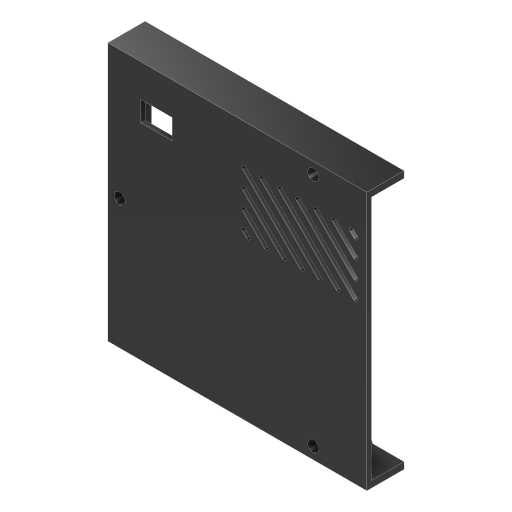
# Autodesk Inventor part: display_cover_part2_back
Saved by Autodesk Inventor 2023 (Build 270158000, 158)
## iProperties
Created: 2024-12-15
Part Number: display_cover_part2_back
Material: Všeobecné
Document SubType Name: Modeling
Designer: Marek
Density: 1 g/cm^3
Appearance: Lesklá – černá
Author: Marek
## iProperties of the stored document display_cover_part2_back_3D tisk.ipt
Created: 2025-01-08
Part Number: display_cover_part2_back_3D tisk
Material: Všeobecné
Document SubType Name: Modeling
Designer: Marek
Density: 1 g/cm^3
Appearance: Výchozí
Author: Marek
Autodesk Inventor part; units mm, degrees
ref_plane "YZ Plane" through (0, 0, 0) normal (1, 0, 0) x (0, 1, 0)
ref_plane "XZ Plane" through (0, 0, 0) normal (0, 1, 0) x (-1, 0, 0)
ref_plane "XY Plane" through (0, 0, 0) normal (0, 0, 1) x (1, 0, 0)
sketch "Náčrt1" plane through (0, 0, 0) normal (0, 0, 1) x (1, 0, 0)
  line L0 (0, 110.95) -> (0, -110.95) projected
  line L1 (-115.25, 0) -> (107, 0) projected
  line L2 (-83.5, 79.25) -> (75.25, 79.25)
  line L3 (75.25, 79.25) -> (75.25, -79.25)
  line L4 (75.25, -79.25) -> (-83.5, -79.25)
  line L5 (-83.5, -79.25) -> (-83.5, 79.25)
  point P0 (0, 0)
  dimension "d0" = 158.75
  dimension "d1" = 158.5
  dimension "d2" = 83.5
  constraints: 8 end point, 2 parallel, 1 horizontal, 1 perpendicular, 1 other
  measures "d0" distance between parallel lines of L5 L3
  measures "d1" distance between parallel lines of L4 L2
  measures "d2" distance between parallel lines of L5 L0
extrude "Vysunutí1" add sketch "Náčrt1" along normal blind 2.8
sketch "Náčrt2" plane through (0, 0, 0) normal (0, 0, -1) x (-1, 0, 0)
  line L0 (0, -110.95) -> (0, 110.95) projected
  line L1 (-107.3, 0) -> (115.3, 0) projected
  line L2 (83.5, -79.25) -> (-75.25, -79.25) projected
  line L3 (83.5, 79.25) -> (83.5, -79.25) projected
  line L4 (-75.25, 79.25) -> (83.5, 79.25) projected
  line L5 (-75.25, -79.25) -> (-75.25, 79.25) projected
  line L6 (-75.25, 75.25) -> (79.5, 75.25)
  line L7 (79.5, 75.25) -> (79.5, -75.25)
  line L8 (79.5, -75.25) -> (-75.25, -75.25)
  line L9 (-75.25, -75.25) -> (-75.25, 75.25)
  line L10 (83.5, -79.25) -> (-75.25, -79.25) projected
  line L11 (-75.25, 79.25) -> (83.5, 79.25)
  line L12 (83.5, 79.25) -> (83.5, -79.25)
  line L13 (83.5, -79.25) -> (-75.25, -79.25)
  line L14 (-75.25, -79.25) -> (-75.25, 79.25)
  line L15 (83.5, 79.25) -> (83.5, -79.25) projected
  arc A0 (79.5, 13.6771) -> (79.5, -13.6771) centre (83.5, 0) ccw
  line L16 (-75.25, 79.25) -> (83.5, 79.25) projected
  arc A1 (-56.0271, 75.25) -> (-28.6729, 75.25) centre (-42.35, 79.25) ccw
  arc A2 (-28.6729, -75.25) -> (-56.0271, -75.25) centre (-42.35, -79.25) ccw
  point P0 (0, 0)
  dimension "d5" = 4
  dimension "d6" = 4
  dimension "d7" = 4
  dimension "d8" = 28.5
  dimension "d9" = 28.5
  dimension "d10" = 28.5
  dimension "d11" = 42.35
  dimension "d12" = 42.35
  constraints: 16 end point, 9 point on line, 6 point on circle, 4 parallel, 3 centre point, 2 horizontal, 2 perpendicular, 1 midpoint
  measures "d5" distance between parallel lines of L4 L6
  measures "d6" distance between parallel lines of L3 L7
  measures "d7" distance between parallel lines of L2 L8
  measures "d8" diameter of A0
  measures "d9" diameter of A1
  measures "d10" diameter of A2
  measures "d11" distance from line of L0 A1.centre
  measures "d12" distance from line of A2.centre L0
extrude "Vysunutí2" add sketch "Náčrt2" along normal blind 20 contours L2 L5 L8 L0 | L0 L8 L7 L1 L3 L2 | L8 A2 | L1 L7 L6 L0 L4 L3 | L6 L5 L4 L0 | A0 L7 L1 | L1 L7 A0 | A1 L6
sketch "Náčrt3" plane through (0, 0, 2.8) normal (0, 0, 1) x (1, 0, 0)
  line L0 (-83.5, -79.25) -> (75.25, -79.25) projected
  line L1 (75.25, -79.25) -> (75.25, 79.25) projected
  line L2 (75.25, 79.25) -> (-83.5, 79.25) projected
  line L3 (-83.5, 79.25) -> (-83.5, -79.25) projected
  line L4 (-115.3, 0) -> (107.3, 0) projected
  line L5 (0, 110.95) -> (0, -110.95) projected
  arc A0 (23.2826, 17.8214) -> (25.4034, 19.9432) centre (24.343, 18.8823) ccw
  line L6 (-1.08, 53.1695) -> (34.2839, 17.8227)
  line L7 (36.4053, 17.8233) -> (-1.0805, 55.2908) construction
  line L8 (36.4047, 19.9446) -> (1.0408, 55.2914)
  arc A1 (34.2839, 17.8227) -> (36.4047, 19.9446) centre (35.3443, 18.8837) ccw
  arc A2 (45.2853, 17.8241) -> (47.4061, 19.9459) centre (46.3457, 18.885) ccw
  line L9 (20.9227, 53.1722) -> (56.2866, 17.8254)
  line L10 (58.4074, 19.9472) -> (23.0435, 55.294)
  line L11 (58.4079, 17.8259) -> (20.9222, 55.2935) construction
  line L12 (31.9396, 53.158) -> (67.0452, 18.0694)
  line L13 (69.166, 20.1912) -> (34.0604, 55.2798)
  line L14 (69.1665, 18.0699) -> (31.9227, 55.2956) construction
  arc A3 (56.2866, 17.8254) -> (58.4074, 19.9472) centre (57.347, 18.8863) ccw
  arc A4 (67.0452, 18.0694) -> (69.166, 20.1912) centre (68.1056, 19.1303) ccw
  line L15 (47.4066, 17.8246) -> (9.9209, 55.2922) construction
  line L16 (9.9214, 53.1709) -> (45.2853, 17.8241)
  arc A5 (12.0422, 55.2927) -> (9.9214, 53.1709) centre (10.9818, 54.2318) ccw
  line L17 (47.4061, 19.9459) -> (12.0422, 55.2927)
  line L18 (53.9267, 53.1762) -> (67.0452, 40.064)
  line L19 (67.2866, 28.8254) -> (42.9254, 53.1748)
  line L20 (69.4079, 28.8259) -> (42.9248, 55.2962) construction
  line L21 (45.0462, 55.2967) -> (69.4074, 30.9472)
  line L22 (69.166, 42.1859) -> (56.0475, 55.298)
  arc A6 (67.2866, 28.8254) -> (69.4074, 30.9472) centre (68.347, 29.8863) ccw
  arc A7 (1.0408, 55.2914) -> (-1.08, 53.1695) centre (-0.0196, 54.2304) ccw
  arc A8 (23.0435, 55.294) -> (20.9227, 53.1722) centre (21.9831, 54.2331) ccw
  line L23 (25.4034, 19.9432) -> (1.0422, 44.2927)
  line L24 (25.4039, 17.8219) -> (-1.0791, 44.2922) construction
  line L25 (-1.0786, 42.1709) -> (23.2826, 17.8214)
  arc A9 (1.0422, 44.2927) -> (-1.0786, 42.1709) centre (-0.0182, 43.2318) ccw
  line L26 (67.2839, 50.8227) -> (64.9396, 53.1659)
  line L27 (67.0604, 55.2878) -> (69.4047, 52.9446)
  line L28 (69.4053, 50.8233) -> (64.9227, 55.3036) construction
  line L29 (69.1665, 40.0645) -> (53.9262, 55.2975) construction
  arc A10 (56.0475, 55.298) -> (53.9267, 53.1762) centre (54.9871, 54.2371) ccw
  arc A11 (12.2813, 17.8201) -> (14.4021, 19.9419) centre (13.3417, 18.881) ccw
  line L30 (14.4021, 19.9419) -> (1.0435, 33.294)
  line L31 (14.4026, 17.8206) -> (-1.0778, 33.2935) construction
  line L32 (-1.0773, 31.1722) -> (12.2813, 17.8201)
  arc A12 (1.0435, 33.294) -> (-1.0773, 31.1722) centre (-0.0169, 32.2331) ccw
  arc A13 (67.2839, 50.8227) -> (69.4047, 52.9446) centre (68.3443, 51.8837) ccw
  arc A14 (45.0462, 55.2967) -> (42.9254, 53.1748) centre (43.9858, 54.2358) ccw
  arc A15 (67.0452, 40.064) -> (69.166, 42.1859) centre (68.1056, 41.125) ccw
  line L33 (1.0448, 22.2953) -> (3.4007, 19.9406)
  arc A16 (1.2799, 17.8187) -> (3.4007, 19.9406) centre (2.3403, 18.8797) ccw
  arc A17 (1.0448, 22.2953) -> (-1.076, 20.1735) centre (-0.0156, 21.2344) ccw
  line L34 (3.4013, 17.8193) -> (-1.0765, 22.2948) construction
  line L35 (1.2799, 17.8187) -> (-1.076, 20.1735)
  arc A18 (34.0604, 55.2798) -> (31.9396, 53.158) centre (33, 54.2189) ccw
  arc A19 (67.0604, 55.2878) -> (64.9396, 53.1659) centre (66, 54.2269) ccw
  point P0 (0, 0)
  dimension "d48" = 3
  dimension "d49" = 3
  dimension "d50" = 3
  dimension "d51" = 3
  dimension "d53" = 3
  dimension "d54" = 3
  dimension "d55" = 3
  dimension "d56" = 3
  dimension "d57" = 3
  dimension "d101" = 23.3345
  dimension "d102" = 31.1127
  dimension "d103" = 38.8909
  dimension "d104" = 46.669
  dimension "d105" = 54.4472
  dimension "d106" = 62.2254
  dimension "d107" = 70.0036
  dimension "d108" = 15.5564
  dimension "d109" = 7.7782
  dimension "d110" = 10.657
  dimension "d131" = 33
  dimension "d132" = 1.5
  dimension "d133" = 66
  dimension "d134" = 1.5
  dimension "d139" = 135.014
  dimension "d140" = 18.5563
  dimension "d141" = 31.1127
  dimension "d142" = 9.157
  dimension "d143" = 1.3789
  dimension "d144" = 50.4241
  dimension "d145" = 28.4267
  dimension "d146" = 39.1855
  dimension "d147" = 23.9464
  dimension "d148" = 61.4254
  dimension "d149" = 61.4267
  dimension "d150" = 23.9544
  dimension "d151" = 61.4281
  dimension "d152" = 61.4294
  dimension "d153" = 23.9573
  dimension "d154" = 61.4307
  dimension "d155" = 56.9547
  dimension "d156" = 45.956
  dimension "d157" = 34.9573
  dimension "d158" = 23.9586
  constraints: 80 end point, 58 point on circle, 37 tangent, 20 centre point, 20 point on line, 12 parallel, 1 equal radius
  measures "d48" distance between parallel lines of L6 L8
  measures "d49" distance between parallel lines of L17 L16
  measures "d50" distance between parallel lines of L25 L23
  measures "d51" distance between parallel lines of L32 L30
  measures "d53" distance between parallel lines of L10 L9
  measures "d54" distance between parallel lines of L12 L13
  measures "d55" distance between parallel lines of L21 L19
  measures "d56" distance between parallel lines of L18 L22
  measures "d57" distance between parallel lines of L26 L27
  measures "d101" distance between parallel lines of L14 L28
  measures "d102" distance between parallel lines of L28 L11
  measures "d103" distance between parallel lines of L28 L15
  measures "d104" distance between parallel lines of L28 L7
  measures "d105" distance between parallel lines of L28 L24
  measures "d106" distance between parallel lines of L28 L31
  measures "d107" distance between parallel lines of L34 L28
  measures "d108" distance between parallel lines of L13 L22
  measures "d109" distance between parallel lines of L29 L20
  measures "d110" distance from line of L4.end L27
  measures "d131" distance from line of L5 A18.centre
  measures "d132" radius of A18
  measures "d133" distance from line of L5 A19.centre
  measures "d134" radius of A19
  measures "d139" angle of L2 L27
  measures "d140" distance between parallel lines of L27 L19
  measures "d141" distance between parallel lines of L27 L10
  measures "d142" distance from line of L4.end L28
  measures "d143" distance from line of L4.end L29
  measures "d144" distance from line of L20.start L2
  measures "d145" distance from line of L28.start L2
  measures "d146" distance from line of L29.start L2
  measures "d147" distance from line of L28.end L2
  measures "d148" distance from line of L15.start L2
  measures "d149" distance from line of L7.start L2
  measures "d150" distance from line of L14.end L2
  measures "d151" distance from line of L24.start L2
  measures "d152" distance from line of L31.start L2
  measures "d153" distance from line of L17.end L2
  measures "d154" distance from line of L34.start L2
  measures "d155" distance from line of L33.start L2
  measures "d156" distance from line of L30.end L2
  measures "d157" distance from line of L23.end L2
  measures "d158" distance from line of L8.end L2
extrude "Vysunutí3" cut sketch "Náčrt3" against normal up to next contours L35 A17 L5 | L5 A17 L33 A16 L35 | A7 L8 A1 L6 L5 | L5 L6 A7 | L32 A12 L5 | L5 A12 L30 A11 L32 | A9 L23 A0 L25 L5 | L5 L25 A9 | L16 A5 L17 A2 | A8 L10 A3 L9 | A18 L13 A4 L12 | A10 L22 A15 L18 | L19 A14 L21 A6 | L26 A19 L27 A13
sketch "Náčrt4" plane through (0, 0, 2.8) normal (0, 0, 1) x (1, 0, 0)
  arc A0 (23.0435, 55.294) -> (20.9227, 53.1722) centre (21.9831, 54.2331) ccw projected
  line L0 (23.0435, 55.294) -> (58.4074, 19.9472) projected
  arc A1 (56.2866, 17.8254) -> (58.4074, 19.9472) centre (57.347, 18.8863) ccw projected
  line L1 (56.2866, 17.8254) -> (20.9227, 53.1722) projected
  arc A2 (67.2839, 50.8227) -> (69.4047, 52.9446) centre (68.3443, 51.8837) ccw projected
  line L2 (67.2839, 50.8227) -> (64.9396, 53.1659) projected
  arc A3 (67.0604, 55.2878) -> (64.9396, 53.1659) centre (66, 54.2269) ccw projected
  line L3 (67.0604, 55.2878) -> (69.4047, 52.9446) projected
  line L4 (1.2799, 17.8187) -> (-1.076, 20.1735) projected
  arc A4 (1.0448, 22.2953) -> (-1.076, 20.1735) centre (-0.0156, 21.2344) ccw projected
  line L5 (1.0448, 22.2953) -> (3.4007, 19.9406) projected
  arc A5 (1.2799, 17.8187) -> (3.4007, 19.9406) centre (2.3403, 18.8797) ccw projected
  arc A6 (56.0475, 55.298) -> (53.9267, 53.1762) centre (54.9871, 54.2371) ccw projected
  line L6 (56.0475, 55.298) -> (69.166, 42.1859) projected
  arc A7 (67.0452, 40.064) -> (69.166, 42.1859) centre (68.1056, 41.125) ccw projected
  line L7 (67.0452, 40.064) -> (53.9267, 53.1762) projected
  arc A8 (12.0422, 55.2927) -> (9.9214, 53.1709) centre (10.9818, 54.2318) ccw projected
  line L8 (12.0422, 55.2927) -> (47.4061, 19.9459) projected
  arc A9 (45.2853, 17.8241) -> (47.4061, 19.9459) centre (46.3457, 18.885) ccw projected
  line L9 (45.2853, 17.8241) -> (9.9214, 53.1709) projected
  arc A10 (34.0604, 55.2798) -> (31.9396, 53.158) centre (33, 54.2189) ccw projected
  line L10 (34.0604, 55.2798) -> (69.166, 20.1912) projected
  arc A11 (67.0452, 18.0694) -> (69.166, 20.1912) centre (68.1056, 19.1303) ccw projected
  line L11 (67.0452, 18.0694) -> (31.9396, 53.158) projected
  line L12 (23.2826, 17.8214) -> (-1.0786, 42.1709) projected
  arc A12 (1.0422, 44.2927) -> (-1.0786, 42.1709) centre (-0.0182, 43.2318) ccw projected
  line L13 (1.0422, 44.2927) -> (25.4034, 19.9432) projected
  arc A13 (23.2826, 17.8214) -> (25.4034, 19.9432) centre (24.343, 18.8823) ccw projected
  line L14 (12.2813, 17.8201) -> (-1.0773, 31.1722) projected
  arc A14 (1.0435, 33.294) -> (-1.0773, 31.1722) centre (-0.0169, 32.2331) ccw projected
  line L15 (1.0435, 33.294) -> (14.4021, 19.9419) projected
  arc A15 (12.2813, 17.8201) -> (14.4021, 19.9419) centre (13.3417, 18.881) ccw projected
  arc A16 (67.2866, 28.8254) -> (69.4074, 30.9472) centre (68.347, 29.8863) ccw projected
  line L16 (67.2866, 28.8254) -> (42.9254, 53.1748) projected
  arc A17 (45.0462, 55.2967) -> (42.9254, 53.1748) centre (43.9858, 54.2358) ccw projected
  line L17 (45.0462, 55.2967) -> (69.4074, 30.9472) projected
  line L18 (34.2839, 17.8227) -> (-1.08, 53.1695) projected
  arc A18 (1.0408, 55.2914) -> (-1.08, 53.1695) centre (-0.0196, 54.2304) ccw projected
  line L19 (1.0408, 55.2914) -> (36.4047, 19.9446) projected
  arc A19 (34.2839, 17.8227) -> (36.4047, 19.9446) centre (35.3443, 18.8837) ccw projected
  line L20 (-83.5, -79.25) -> (75.25, -79.25) projected
  line L21 (75.25, -79.25) -> (75.25, 79.25) projected
  line L22 (75.25, 79.25) -> (-83.5, 79.25) projected
  line L23 (-83.5, 79.25) -> (-83.5, -79.25) projected
  line L24 (0, 110.95) -> (0, -110.95) projected
  line L25 (-115.25, 0) -> (107, 0) projected
  arc A20 (28.6729, 75.25) -> (56.0271, 75.25) centre (42.35, 79.25) ccw projected
  arc A21 (-79.5, -13.6771) -> (-79.5, 13.6771) centre (-83.5, 0) ccw projected
  arc A22 (56.0271, -75.25) -> (28.6729, -75.25) centre (42.35, -79.25) ccw projected
  point P0 (0, 0)
  point P1 (42.35, 72.125)
  point P2 (-76.375, 0)
  point P3 (42.35, -72.125)
  dimension "d159" = 7.125
  dimension "d160" = 42.35
  dimension "d161" = 7.125
  dimension "d162" = 42.35
  dimension "d163" = 7.125
  constraints: 1 point on line
  measures "d159" distance from line of point (42.35, 72.125) L22
  measures "d160" distance from line of L24 point (42.35, 72.125)
  measures "d161" distance from line of L20 point (42.35, -72.125)
  measures "d162" distance from line of L24 point (42.35, -72.125)
  measures "d163" distance from line of L23 point (-76.375, 0)
hole "Díra1" at (42.35, 72.125, 2.8) at (-76.375, 0, 2.8) at (42.35, -72.125, 2.8) direction (0, 0, -1) diameter 7 depth 6
sketch "Náčrt5" plane through (42.35, 72.125, -3.2) normal (0, 0, 1) x (1, 0, 0)
  circle A0 centre (0, 0) radius 3.5 projected
  circle A1 centre (-118.725, -72.125) radius 3.5 projected
  circle A2 centre (0, -144.25) radius 3.5 projected
  circle A3 centre (0, 0) radius 3.5 projected
  circle A4 centre (0, -144.25) radius 3.5 projected
  point P0 (-42.35, -72.125)
  constraints: 3 coincident
hole "Díra2" at (-76.375, 0, -3.2) at (42.35, 72.125, -3.2) at (42.35, -72.125, -3.2) direction (0, 0, -1) diameter 3.4 depth 16.8
sketch "Náčrt6" plane through (0, 0, 2.8) normal (0, 0, 1) x (1, 0, 0)
  line L0 (0, 110.95) -> (0, -110.95) projected
  line L1 (-115.25, 0) -> (107, 0) projected
  circle A0 centre (-76.375, 0) radius 3.5 projected
  circle A1 centre (42.35, 72.125) radius 3.5 projected
  circle A2 centre (42.35, -72.125) radius 3.5 projected
  arc A3 (23.0435, 55.294) -> (20.9227, 53.1722) centre (21.9831, 54.2331) ccw projected
  line L2 (23.0435, 55.294) -> (58.4074, 19.9472) projected
  arc A4 (56.2866, 17.8254) -> (58.4074, 19.9472) centre (57.347, 18.8863) ccw projected
  line L3 (56.2866, 17.8254) -> (20.9227, 53.1722) projected
  arc A5 (67.2839, 50.8227) -> (69.4047, 52.9446) centre (68.3443, 51.8837) ccw projected
  line L4 (67.2839, 50.8227) -> (64.9396, 53.1659) projected
  arc A6 (67.0604, 55.2878) -> (64.9396, 53.1659) centre (66, 54.2269) ccw projected
  line L5 (67.0604, 55.2878) -> (69.4047, 52.9446) projected
  line L6 (1.2799, 17.8187) -> (-1.076, 20.1735) projected
  arc A7 (1.0448, 22.2953) -> (-1.076, 20.1735) centre (-0.0156, 21.2344) ccw projected
  line L7 (1.0448, 22.2953) -> (3.4007, 19.9406) projected
  arc A8 (1.2799, 17.8187) -> (3.4007, 19.9406) centre (2.3403, 18.8797) ccw projected
  arc A9 (56.0475, 55.298) -> (53.9267, 53.1762) centre (54.9871, 54.2371) ccw projected
  line L8 (56.0475, 55.298) -> (69.166, 42.1859) projected
  arc A10 (67.0452, 40.064) -> (69.166, 42.1859) centre (68.1056, 41.125) ccw projected
  line L9 (67.0452, 40.064) -> (53.9267, 53.1762) projected
  arc A11 (12.0422, 55.2927) -> (9.9214, 53.1709) centre (10.9818, 54.2318) ccw projected
  line L10 (12.0422, 55.2927) -> (47.4061, 19.9459) projected
  arc A12 (45.2853, 17.8241) -> (47.4061, 19.9459) centre (46.3457, 18.885) ccw projected
  line L11 (45.2853, 17.8241) -> (9.9214, 53.1709) projected
  arc A13 (34.0604, 55.2798) -> (31.9396, 53.158) centre (33, 54.2189) ccw projected
  line L12 (34.0604, 55.2798) -> (69.166, 20.1912) projected
  arc A14 (67.0452, 18.0694) -> (69.166, 20.1912) centre (68.1056, 19.1303) ccw projected
  line L13 (67.0452, 18.0694) -> (31.9396, 53.158) projected
  line L14 (23.2826, 17.8214) -> (-1.0786, 42.1709) projected
  arc A15 (1.0422, 44.2927) -> (-1.0786, 42.1709) centre (-0.0182, 43.2318) ccw projected
  line L15 (1.0422, 44.2927) -> (25.4034, 19.9432) projected
  arc A16 (23.2826, 17.8214) -> (25.4034, 19.9432) centre (24.343, 18.8823) ccw projected
  line L16 (12.2813, 17.8201) -> (-1.0773, 31.1722) projected
  arc A17 (1.0435, 33.294) -> (-1.0773, 31.1722) centre (-0.0169, 32.2331) ccw projected
  line L17 (1.0435, 33.294) -> (14.4021, 19.9419) projected
  arc A18 (12.2813, 17.8201) -> (14.4021, 19.9419) centre (13.3417, 18.881) ccw projected
  arc A19 (67.2866, 28.8254) -> (69.4074, 30.9472) centre (68.347, 29.8863) ccw projected
  line L18 (67.2866, 28.8254) -> (42.9254, 53.1748) projected
  arc A20 (45.0462, 55.2967) -> (42.9254, 53.1748) centre (43.9858, 54.2358) ccw projected
  line L19 (45.0462, 55.2967) -> (69.4074, 30.9472) projected
  line L20 (34.2839, 17.8227) -> (-1.08, 53.1695) projected
  arc A21 (1.0408, 55.2914) -> (-1.08, 53.1695) centre (-0.0196, 54.2304) ccw projected
  line L21 (1.0408, 55.2914) -> (36.4047, 19.9446) projected
  arc A22 (34.2839, 17.8227) -> (36.4047, 19.9446) centre (35.3443, 18.8837) ccw projected
  line L22 (-83.5, -79.25) -> (75.25, -79.25) projected
  line L23 (75.25, -79.25) -> (75.25, 79.25) projected
  line L24 (75.25, 79.25) -> (-83.5, 79.25) projected
  line L25 (-83.5, 79.25) -> (-83.5, -79.25) projected
  line L26 (-63.5, 59.25) -> (-44.1, 59.25)
  line L27 (-44.1, 59.25) -> (-44.1, 46.75)
  line L28 (-44.1, 46.75) -> (-63.5, 46.75)
  line L29 (-63.5, 46.75) -> (-63.5, 59.25)
  point P0 (0, 0)
  dimension "d178" = 19.4
  dimension "d179" = 12.5
  dimension "d180" = 20
  dimension "d181" = 20
  constraints: 8 end point, 2 parallel, 1 horizontal, 1 perpendicular
  measures "d178" distance between parallel lines of L29 L27
  measures "d179" distance between parallel lines of L28 L26
  measures "d180" distance between parallel lines of L25 L29
  measures "d181" distance between parallel lines of L24 L26
extrude "Vysunutí4" cut sketch "Náčrt6" against normal up to surface (2.8 mm away) contours L26 L27 L28 L29
sketch "Náčrt7" plane through (0, 0, 0) normal (0, 0, -1) x (-1, 0, 0)
  line L0 (0, -110.95) -> (0, 110.95) projected
  line L1 (-107, 0) -> (115.25, 0) projected
  line L2 (-50, 12.75) -> (-40, 12.75)
  line L3 (-40, 12.75) -> (-40, 5.75)
  line L4 (-40, 5.75) -> (-50, 5.75)
  line L5 (-50, 5.75) -> (-50, 12.75)
  line L6 (-50, -55.25) -> (-40, -55.25)
  line L7 (-40, -55.25) -> (-40, -62.25)
  line L8 (-40, -62.25) -> (-50, -62.25)
  line L9 (-50, -62.25) -> (-50, -55.25)
  line L10 (35, 12.75) -> (45, 12.75)
  line L11 (45, 12.75) -> (45, 5.75)
  line L12 (45, 5.75) -> (35, 5.75)
  line L13 (35, 5.75) -> (35, 12.75)
  line L14 (35, -55.25) -> (45, -55.25)
  line L15 (45, -55.25) -> (45, -62.25)
  line L16 (45, -62.25) -> (35, -62.25)
  line L17 (35, -62.25) -> (35, -55.25)
  line L18 (79.5, -75.25) -> (-28.6729, -75.25) projected
  point P0 (0, 0)
  point P1 (35, -58.75)
  dimension "d184" = 61
  dimension "d185" = 13
  dimension "d186" = 7
  dimension "d187" = 10
  dimension "d188" = 7
  dimension "d189" = 10
  dimension "d190" = 40
  dimension "d191" = 40
  dimension "d192" = 35
  dimension "d193" = 35
  dimension "d194" = 61
  dimension "d195" = 13
  dimension "d196" = 7
  dimension "d197" = 10
  dimension "d198" = 7
  constraints: 32 end point, 8 parallel, 4 horizontal, 4 perpendicular, 1 midpoint, 1 point on line
  measures "d184" distance between parallel lines of L6 L4
  measures "d185" distance between parallel lines of L18 L8
  measures "d186" distance between parallel lines of L8 L6
  measures "d187" distance between parallel lines of L9 L7
  measures "d188" distance between parallel lines of L2 L4
  measures "d189" distance between parallel lines of L5 L3
  measures "d190" distance between parallel lines of L7 L0
  measures "d191" distance between parallel lines of L0 L3
  measures "d192" distance between parallel lines of L0 L13
  measures "d193" distance between parallel lines of L0 L17
  measures "d194" distance between parallel lines of L14 L12
  measures "d195" distance between parallel lines of L18 L16
  measures "d196" distance between parallel lines of L16 L14
  measures "d197" distance from line of point (35, -58.75) L15
  measures "d198" distance between parallel lines of L10 L12
extrude "Vysunutí5" add sketch "Náčrt7" along normal blind 13.5
sketch "Náčrt8" plane through (0, 0, -13.5) normal (0, 0, -1) x (-1, 0, 0)
  line L0 (-50, 5.75) -> (-40, 5.75) projected
  line L1 (-40, 5.75) -> (-40, 12.75) projected
  line L2 (-40, 12.75) -> (-50, 12.75) projected
  line L3 (-50, 12.75) -> (-50, 5.75) projected
  line L4 (35, 5.75) -> (45, 5.75) projected
  line L5 (45, 5.75) -> (45, 12.75) projected
  line L6 (45, 12.75) -> (35, 12.75) projected
  line L7 (35, 12.75) -> (35, 5.75) projected
  line L8 (35, -62.25) -> (45, -62.25) projected
  line L9 (45, -62.25) -> (45, -55.25) projected
  line L10 (45, -55.25) -> (35, -55.25) projected
  line L11 (35, -55.25) -> (35, -62.25) projected
  line L12 (-50, -62.25) -> (-40, -62.25) projected
  line L13 (-40, -62.25) -> (-40, -55.25) projected
  line L14 (-40, -55.25) -> (-50, -55.25) projected
  line L15 (-50, -55.25) -> (-50, -62.25) projected
  point P0 (0, 0)
  point P1 (-45, 9.25)
  point P2 (40, 9.25)
  point P3 (40, -58.75)
  point P4 (-45, -58.75)
  point P5 (40, 5.75)
  dimension "d202" = 5
  dimension "d204" = 5
  dimension "d206" = 5
  dimension "d207" = 5
  dimension "d216" = 3.5
  dimension "d217" = 3.5
  dimension "d218" = 3.5
  dimension "d219" = 3.5
  constraints: 1 midpoint
  measures "d202" distance from line of L1 point (-45, 9.25)
  measures "d204" distance from line of L7 point (40, 9.25)
  measures "d206" distance from line of point (40, -58.75) L11
  measures "d207" distance from line of point (-45, -58.75) L13
  measures "d216" distance from line of L0 point (-45, 9.25)
  measures "d217" distance from line of L4 point (40, 9.25)
  measures "d218" distance from line of L8 point (40, -58.75)
  measures "d219" distance from line of L12 point (-45, -58.75)
hole "Díra3" at (45, 9.25, -13.5) at (-40, 9.25, -13.5) at (-40, -58.75, -13.5) at (45, -58.75, -13.5) direction (0, 0, 1) diameter 2.1 depth 11 tip angle 118
equation "\"d49\" = d48"
equation "\"d50\" = d48"
equation "\"d51\" = d48"
equation "\"d53\" = d48"
equation "\"d54\" = d48"
equation "\"d55\" = d48"
equation "\"d56\" = d48"
equation "\"d57\" = d49"
